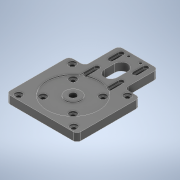
# Autodesk Inventor part: Shoulderbasetop
Saved by Autodesk Inventor 2022 (Build 260153000, 153)
## iProperties
Created: 2022-03-24
Part Number: Shoulderbasetop
Material: Genérico
Document SubType Name: Modeling
Designer: JK
Density: 1 g/cm^3
Appearance: Suave - Negro
Author: JK
Autodesk Inventor part; units mm, degrees
ref_plane "YZ Plane" through (0, 0, 0) normal (1, 0, 0) x (0, 1, 0)
ref_plane "XZ Plane" through (0, 0, 0) normal (0, 1, 0) x (-1, 0, 0)
ref_plane "XY Plane" through (0, 0, 0) normal (0, 0, 1) x (1, 0, 0)
sketch "Boceto1" plane through (0, 0, 0) normal (0, 1, 0) x (-1, 0, 0)
  circle A0 centre (0, 0) radius 4.35
  line L0 (-45, 40) -> (45, 40)
  line L1 (45, 40) -> (45, -40)
  line L2 (45, -40) -> (-45, -40)
  line L3 (-45, -40) -> (-45, 40)
  line L4 (-45, 40) -> (45, -40) construction
  line L5 (45, 40) -> (-45, -40) construction
  dimension "d0" = 8.7
  dimension "d1" = 80
  dimension "d2" = 90
  constraints: 12 end point, 2 midpoint, 2 parallel, 1 centre point, 1 coincident, 1 horizontal, 1 perpendicular
  measures "d0" diameter of A0
  measures "d1" distance of L0.end L1.end
  measures "d2" distance of L1.end L2.end
extrude "Extrusión1" add sketch "Boceto1" along normal blind 10
sketch "Boceto2" plane through (0, 10, 0) normal (0, 1, 0) x (1, 0, 0)
  circle A0 centre (0, 0) radius 4.35 projected
  circle A1 centre (0, 0) radius 32.875
  dimension "d5" = 65.75
  constraints: 1 centre point, 1 coincident
  measures "d5" diameter of A1
extrude "Extrusión2" cut sketch "Boceto2" against normal blind 1.4
sketch "Boceto3" plane through (0, 8.6, 0) normal (0, 1, 0) x (1, 0, 0)
  circle A0 centre (0, 0) radius 4.35 projected
  circle A1 centre (0, 0) radius 10
  dimension "d8" = 20
  constraints: 1 centre point, 1 coincident
  measures "d8" diameter of A1
extrude "Extrusión3" add sketch "Boceto3" along normal up to surface (1.4 mm away)
sketch "Boceto4" plane through (0, 8.6, 0) normal (0, 1, 0) x (1, 0, 0)
  circle A0 centre (0, -18.25) radius 2.65
  circle A1 centre (0, 18.25) radius 2.65
  point P0 (0, 0)
  dimension "d11" = 5.3
  dimension "d12" = 36.5
  dimension "d13" = 18.25
  constraints: 2 centre point, 1 equal radius
  measures "d11" diameter of A0
  measures "d12" distance of A1.centre A0.centre
  measures "d13" distance of A1.centre point (0, 0)
extrude "Extrusión4" [suppressed]
sketch "Boceto5" plane through (0, 8.6, 0) normal (0, 1, 0) x (1, 0, 0)
  circle A0 centre (0, -18.25) radius 2.65 projected
  circle A1 centre (0, -18.25) radius 4.05
  circle A2 centre (0, 18.25) radius 2.65 projected
  circle A3 centre (0, 18.25) radius 4.05
  line L0 (-4.6765, -18.25) -> (-2.3383, -14.2)
  line L1 (-2.3383, -14.2) -> (2.3383, -14.2)
  line L2 (2.3383, -14.2) -> (4.6765, -18.25)
  line L3 (4.6765, -18.25) -> (2.3383, -22.3)
  line L4 (2.3383, -22.3) -> (-2.3383, -22.3)
  line L5 (-2.3383, -22.3) -> (-4.6765, -18.25)
  line L6 (-4.6765, 18.25) -> (-2.3383, 22.3)
  line L7 (-2.3383, 22.3) -> (2.3383, 22.3)
  line L8 (2.3383, 22.3) -> (4.6765, 18.25)
  line L9 (4.6765, 18.25) -> (2.3383, 14.2)
  line L10 (2.3383, 14.2) -> (-2.3383, 14.2)
  line L11 (-2.3383, 14.2) -> (-4.6765, 18.25)
  point P0 (0, 0)
  dimension "d16" = 8.1
  constraints: 24 end point, 4 coincident, 2 centre point, 2 horizontal, 2 tangent, 1 equal radius, 26 other
  measures "d16" diameter of A1
extrude "Extrusión5" [suppressed]
sketch "Boceto6" plane through (0, 10, 0) normal (0, 1, 0) x (1, 0, 0)
  circle A0 centre (-35, 34) radius 2.7
  circle A1 centre (35, 34) radius 2.7
  circle A2 centre (-35, -34) radius 2.7
  circle A3 centre (35, -34) radius 2.7
  line L0 (-45, 40) -> (-45, -40) projected
  line L1 (45, 40) -> (-45, 40) projected
  line L2 (-45, -40) -> (45, -40) projected
  line L3 (45, -40) -> (45, 40) projected
  point P0 (0, 0)
  dimension "d19" = 5.4
  dimension "d20" = 10
  dimension "d21" = 6
  dimension "d22" = 6
  dimension "d23" = 10
  constraints: 4 centre point, 3 equal radius, 2 horizontal alignment, 2 vertical alignment
  measures "d19" diameter of A0
  measures "d20" distance from line of L0 A0.centre
  measures "d21" distance from line of L1 A0.centre
  measures "d22" distance from line of A2.centre L2
  measures "d23" distance from line of L3 A1.centre
extrude "Extrusión6" cut sketch "Boceto6" against normal through all contours A0 | A1 | A2 | A3
fillet "Empalme1" radius 5 4 edges at (45, 5, 40) (45, 5, -40) (-45, 5, 40) (-45, 5, -40)
sketch "Boceto7" plane through (0, 10, 0) normal (0, 1, 0) x (1, 0, 0)
  circle A0 centre (-35, -34) radius 2.7 projected
  circle A1 centre (-35, -34) radius 4.7
  circle A2 centre (35, -34) radius 2.7 projected
  circle A3 centre (35, -34) radius 4.7
  circle A4 centre (35, 34) radius 2.7 projected
  circle A5 centre (35, 34) radius 4.7
  circle A6 centre (-35, 34) radius 2.7 projected
  circle A7 centre (-35, 34) radius 4.7
  point P0 (0, 0)
  dimension "d27" = 9.4
  constraints: 4 centre point, 4 coincident, 3 equal radius
  measures "d27" diameter of A7
extrude "Extrusión7" cut sketch "Boceto7" against normal blind 2.1 contours A0 | A1 | A2 | A3 | A4 | A5 | A6 | A7
sketch "Boceto9" plane through (0, 0, 0) normal (0, -1, 0) x (1, 0, 0)
  circle A0 centre (0, 0) radius 4.35 projected
  circle A1 centre (0, 0) radius 8.125
  dimension "d32" = 16.25
  constraints: 1 centre point, 1 coincident
  measures "d32" diameter of A1
extrude "Extrusión9" cut sketch "Boceto9" against normal blind 5 contours A0 | A1
sketch "Boceto10" plane through (0, 8.6, 0) normal (0, 1, 0) x (1, 0, 0)
  circle A0 centre (19, -19) radius 2.7
  line L0 (26, 26) -> (-26, 26)
  line L1 (-26, 26) -> (-26, -26)
  line L2 (-26, -26) -> (26, -26)
  line L3 (26, -26) -> (26, 26)
  circle A1 centre (0, 0) radius 4.35 projected
  line L4 (26, 26) -> (-26, -26) construction
  line L5 (-26, 26) -> (26, -26) construction
  circle A2 centre (0, 0) radius 10 projected
  circle A3 centre (0, 0) radius 21
  circle A4 centre (19, -19) radius 5
  line L6 (-19, 19) -> (19, 19)
  line L7 (19, 19) -> (19, -19)
  line L8 (19, -19) -> (-19, -19)
  line L9 (-19, -19) -> (-19, 19)
  line L10 (-19, 19) -> (19, -19) construction
  line L11 (19, 19) -> (-19, -19) construction
  dimension "d35" = 52
  dimension "d36" = 52
  dimension "d37" = 42
  dimension "d38" = 5.4
  dimension "d39" = 10
  dimension "d40" = 38
  constraints: 24 end point, 4 midpoint, 4 parallel, 3 centre point, 2 coincident, 2 horizontal, 2 perpendicular, 1 point on line
  measures "d35" distance of L2.end L1.end
  measures "d36" distance of L0.end L1.end
  measures "d37" diameter of A3
  measures "d38" diameter of A0
  measures "d39" diameter of A4
  measures "d40" distance of L7.end L8.end
extrude "Extrusión10" cut sketch "Boceto10" against normal through all contours A0 L8 L7 | L7 L8 A0
sketch "Boceto11" plane through (0, 8.6, 0) normal (0, 1, 0) x (1, 0, 0)
  circle A0 centre (19, -19) radius 2.7 projected
  circle A1 centre (19, -19) radius 4.7
  point P0 (0, 0)
  dimension "d43" = 9.4
  constraints: 1 centre point, 1 coincident
  measures "d43" diameter of A1
extrude "Extrusión11" cut sketch "Boceto11" against normal blind 2.3
pattern_circular "Patrón circular1" count 4 over 360 about axis through (0, 8.6, 0) along (0, 1, 0) of "Extrusión10", "Extrusión11"
sketch "Boceto12" plane through (0, 10, 0) normal (0, 1, 0) x (1, 0, 0)
  line L0 (40, 40) -> (-40, 40) projected
  line L1 (25, 40) -> (-25, 40)
  line L2 (-25, 40) -> (-25, 83)
  line L3 (-25, 83) -> (25, 83)
  line L4 (25, 83) -> (25, 40)
  point P0 (0, 0)
  point P1 (-25, 40)
  dimension "d49" = 25
  dimension "d50" = 25
  dimension "d51" = 43
  constraints: 8 end point, 2 parallel, 1 horizontal, 1 perpendicular, 1 point on line
  measures "d49" distance from line of point (0, 0) L4
  measures "d50" distance from line of point (0, 0) L2
  measures "d51" distance between parallel lines of L0 L3
extrude "Extrusión12" add sketch "Boceto12" against normal up to surface (10 mm away)
fillet "Empalme2" radius 5 4 edges at (25, 5, -40) (25, 5, -83) (-25, 5, -83) (-25, 5, -40)
sketch "Boceto13" plane through (0, 10, 0) normal (0, 1, 0) x (1, 0, 0)
  circle A0 centre (0, 48) radius 8.5
  circle A1 centre (0, 61) radius 8.5
  line L0 (-8.5, 48) -> (8.5, 48)
  line L1 (8.5, 48) -> (8.5, 61)
  line L2 (8.5, 61) -> (-8.5, 61)
  line L3 (-8.5, 61) -> (-8.5, 48)
  line L4 (20, 83) -> (-20, 83) projected
  point P0 (0, 0)
  dimension "d55" = 17
  dimension "d57" = 13
  dimension "d93" = 48
  constraints: 8 end point, 3 vertical, 2 parallel, 1 horizontal, 1 perpendicular, 6 other
  measures "d57" distance of L2.end L0.start
  measures "d93" distance of point (0, 0) point (0, 48)
extrude "Extrusión13" cut sketch "Boceto13" against normal through all
sketch "Boceto14" plane through (0, 10, 0) normal (0, 1, 0) x (1, 0, 0)
  circle A0 centre (-15.5, 32.5) radius 1.7
  line L0 (-17.2, 32.5) -> (-13.8, 32.5)
  line L1 (-13.8, 32.5) -> (-13.8, 45.5)
  line L2 (-13.8, 45.5) -> (-17.2, 45.5)
  line L3 (-17.2, 45.5) -> (-17.2, 32.5)
  circle A1 centre (-15.5, 45.5) radius 1.7
  arc A2 (-8.5, 48) -> (8.5, 48) centre (0, 48) ccw projected
  line L4 (0, 48) -> (-15.5, 48)
  line L5 (-15.5, 48) -> (-15.5, 32.5)
  line L6 (-15.5, 32.5) -> (0, 32.5)
  line L7 (0, 32.5) -> (0, 48)
  point P0 (0, 0)
  point P1 (-13.8, 45.5)
  dimension "d62" = 3.4
  dimension "d60" = 15.5
  dimension "d61" = 15.5
  dimension "d63" = 13
  constraints: 16 end point, 4 parallel, 3 vertical, 2 horizontal, 2 perpendicular, 1 midpoint, 6 other
  measures "d60" distance of L4.end L5.end
  measures "d61" distance of L5.end L6.end
  measures "d63" distance of L2.end L0.start
extrude "Extrusión14" cut sketch "Boceto14" against normal through all contours L0 A0 | L3 A1 L5 A0 | A0 L5 L0 | L0 L5 A0 | A0 L5 A1 L1 | A1 L5 L2 | L2 L5 A1 | A1 L5 L2 | L2 L5 A1
pattern_linear "Patrón rectangular1" count 2 spacing 31 along (0, 0, -1) count 2 spacing 31 along (1, 0, 0) of "Extrusión14"
sketch "Boceto15" plane through (0, 10, 0) normal (0, 1, 0) x (1, 0, 0)
  arc A0 (-17.2, 32.5) -> (-13.8, 32.5) centre (-15.5, 32.5) ccw projected
  line L0 (-17.2, 32.5) -> (-17.2, 45.5) projected
  line L1 (-13.8, 45.5) -> (-13.8, 32.5) projected
  arc A1 (-13.8, 45.5) -> (-17.2, 45.5) centre (-15.5, 45.5) ccw projected
  line L2 (-18.7, 45.5) -> (-18.7, 32.5)
  arc A2 (-18.7, 32.5) -> (-12.3, 32.5) centre (-15.5, 32.5) ccw
  line L3 (-12.3, 32.5) -> (-12.3, 45.5)
  arc A3 (-12.3, 45.5) -> (-18.7, 45.5) centre (-15.5, 45.5) ccw
  point P0 (0, 0)
  point P1 (-17.2, 28.0165)
  point P2 (-13.8, 29.8383)
  dimension "d72" = 1.5
  constraints: 4 end point, 4 point on circle, 2 centre point, 3 other
  measures "d72" distance between parallel lines of L0 L2
extrude "Extrusión15" cut sketch "Boceto15" against normal blind 3 contours L0 A1 L1 A0 | A3 L3 A2 L2
pattern_linear "Patrón rectangular2" count 2 spacing 31 along (0, 0, -1) count 2 spacing 31 along (1, 0, 0) of "Extrusión15"
sketch "Boceto16" plane through (0, 10, 0) normal (0, 1, 0) x (1, 0, 0)
  circle A0 centre (-7.5, 78) radius 1.7
  circle A1 centre (7.5, 78) radius 1.7
  arc A2 (8.5, 61) -> (-8.5, 61) centre (0, 61) ccw projected
  line L0 (20, 83) -> (-20, 83) projected
  point P0 (0, 0)
  dimension "d81" = 3.4
  dimension "d82" = 15
  dimension "d83" = 7.5
  dimension "d84" = 5
  constraints: 2 centre point, 1 equal radius, 1 horizontal alignment
  measures "d81" diameter of A0
  measures "d82" distance of A1.centre A0.centre
  measures "d83" horizontal distance of A2.centre A1.centre
  measures "d84" distance from line of L0 A0.centre
extrude "Extrusión16" cut sketch "Boceto16" against normal through all
sketch "Boceto17" plane through (0, 0, 0) normal (0, -1, 0) x (1, 0, 0)
  circle A0 centre (-7.5, -78) radius 1.7 projected
  circle A1 centre (-7.5, -78) radius 2.85
  circle A2 centre (7.5, -78) radius 1.7 projected
  circle A3 centre (7.5, -78) radius 2.85
  line L0 (-4.2091, -78) -> (-5.8546, -80.85)
  line L1 (-5.8546, -80.85) -> (-9.1454, -80.85)
  line L2 (-9.1454, -80.85) -> (-10.7909, -78)
  line L3 (-10.7909, -78) -> (-9.1454, -75.15)
  line L4 (-9.1454, -75.15) -> (-5.8546, -75.15)
  line L5 (-5.8546, -75.15) -> (-4.2091, -78)
  line L6 (10.7909, -78) -> (9.1454, -80.85)
  line L7 (9.1454, -80.85) -> (5.8546, -80.85)
  line L8 (5.8546, -80.85) -> (4.2091, -78)
  line L9 (4.2091, -78) -> (5.8546, -75.15)
  line L10 (5.8546, -75.15) -> (9.1454, -75.15)
  line L11 (9.1454, -75.15) -> (10.7909, -78)
  point P0 (0, 0)
  dimension "d87" = 5.7
  constraints: 24 end point, 4 coincident, 2 centre point, 2 horizontal, 2 tangent, 1 equal radius, 26 other
  measures "d87" diameter of A1
extrude "Extrusión17" cut sketch "Boceto17" against normal blind 3.1 contours A0 | A1 | A1 L5 L0 | A1 L4 L5 | L0 L1 A1 | A1 L3 L4 | L1 L2 A1 | A1 L2 L3 | A2 | A3 | A3 L11 L6 | A3 L10 L11 | L6 L7 A3 | A3 L9 L10 | L7 L8 A3 | A3 L8 L9
sketch "Boceto18" plane through (0, 10, 0) normal (0, 1, 0) x (1, 0, 0)
  line L0 (-18.7, 32.5) -> (-18.7, 45.5) projected
  line L1 (-18.7, 32.5) -> (-12.3, 32.5)
  line L2 (-12.3, 32.5) -> (-12.3, 25.1645)
  line L3 (-12.3, 25.1645) -> (-18.7, 25.1645)
  line L4 (-18.7, 25.1645) -> (-18.7, 32.5)
  line L5 (12.3, 32.5) -> (12.3, 45.5) projected
  line L6 (12.3, 32.5) -> (18.7, 32.5)
  line L7 (18.7, 32.5) -> (18.7, 9.5036)
  line L8 (18.7, 9.5036) -> (12.3, 9.5036)
  line L9 (12.3, 9.5036) -> (12.3, 32.5)
  line L10 (18.7, 45.5) -> (18.7, 32.5) projected
  line L11 (-12.3, 45.5) -> (-12.3, 32.5) projected
  point P0 (0, 0)
  constraints: 16 end point, 4 parallel, 2 collinear, 2 horizontal, 2 perpendicular
extrude "Extrusión18" cut sketch "Boceto18" against normal up to surface (1.4 mm away)
sketch "Boceto8" plane through (0, 10, 0) normal (0, 1, 0) x (1, 0, 0)
  line L0 (4.981, 25.0262) -> (-4.981, 25.0262)
  line L1 (-4.981, 25.0262) -> (-4.981, 54.9738)
  line L2 (-4.981, 54.9738) -> (4.981, 54.9738)
  line L3 (4.981, 54.9738) -> (4.981, 25.0262)
  line L4 (40, 40) -> (-40, 40) projected
  line L5 (4.981, 25.0262) -> (-4.981, 54.9738) construction
  line L6 (-4.981, 25.0262) -> (4.981, 54.9738) construction
  point P0 (0, 0)
  point P1 (0, 40)
  constraints: 12 end point, 3 midpoint, 2 parallel, 1 horizontal, 1 perpendicular
